Autodesk Inventor part; units mm, degrees
(part 2 of 2)
  line L937 (28.6172, -1.9519) -> (28.5556, -1.9543)
  line L938 (28.5556, -1.9543) -> (28.5008, -1.9651)
  line L939 (28.5008, -1.9651) -> (28.4534, -1.9836)
  line L940 (28.4534, -1.9836) -> (28.4139, -2.0092)
  line L941 (28.4139, -2.0092) -> (28.3764, -2.0503)
  line L942 (28.3764, -2.0503) -> (28.2958, -2.1772)
  line L943 (28.2958, -2.1772) -> (28.1956, -2.3218)
  line L944 (28.1956, -2.3218) -> (28.0891, -2.4618)
  line L945 (28.0891, -2.4618) -> (27.9933, -2.5776)
  line L946 (27.9933, -2.5776) -> (27.9658, -2.626)
  line L947 (27.9658, -2.626) -> (27.9536, -2.6714)
  line L948 (27.9536, -2.6714) -> (27.9506, -2.7222)
  line L949 (27.9506, -2.7222) -> (27.9573, -2.7777)
  line L950 (27.9573, -2.7777) -> (27.974, -2.837)
  line L951 (27.974, -2.837) -> (28.001, -2.8995)
  line L952 (28.001, -2.8995) -> (28.0386, -2.9643)
  line L953 (28.0386, -2.9643) -> (28.0871, -3.0308)
  line L954 (28.0871, -3.0308) -> (28.1466, -3.098)
  line L955 (28.1466, -3.098) -> (28.2172, -3.1653)
  line L956 (28.2172, -3.1653) -> (28.2991, -3.2317)
  line L957 (28.2991, -3.2317) -> (28.3923, -3.2964)
  line L958 (28.3923, -3.2964) -> (28.4154, -3.3262)
  line L959 (28.4154, -3.3262) -> (28.4622, -3.3971)
  line L960 (28.4622, -3.3971) -> (28.5192, -3.5016)
  line L961 (28.5192, -3.5016) -> (28.5791, -3.6371)
  line L962 (28.5791, -3.6371) -> (28.6102, -3.7211)
  line L963 (28.6102, -3.7211) -> (28.6391, -3.8103)
  line L964 (28.6391, -3.8103) -> (28.6674, -3.912)
  line L965 (28.6674, -3.912) -> (28.6928, -4.0208)
  line L966 (28.6928, -4.0208) -> (28.7153, -4.1393)
  line L967 (28.7153, -4.1393) -> (28.734, -4.2669)
  line L968 (28.734, -4.2669) -> (28.7482, -4.4039)
  line L969 (28.7482, -4.4039) -> (28.7571, -4.5485)
  line L970 (28.7571, -4.5485) -> (28.7599, -4.6757)
  arc A19 (28.2849, -5.0208) -> (28.7599, -4.6757) centre (25, 0) ccw
  line L971 (28.2849, -5.0208) -> (28.1648, -4.9789)
  line L972 (28.1648, -4.9789) -> (28.0301, -4.9258)
  line L973 (28.0301, -4.9258) -> (27.9042, -4.8699)
  line L974 (27.9042, -4.8699) -> (27.7886, -4.8127)
  line L975 (27.7886, -4.8127) -> (27.6829, -4.7547)
  line L976 (27.6829, -4.7547) -> (27.5872, -4.697)
  line L977 (27.5872, -4.697) -> (27.4992, -4.6386)
  line L978 (27.4992, -4.6386) -> (27.4233, -4.5836)
  line L979 (27.4233, -4.5836) -> (27.353, -4.528)
  line L980 (27.353, -4.528) -> (27.2426, -4.4291)
  line L981 (27.2426, -4.4291) -> (27.1609, -4.3427)
  line L982 (27.1609, -4.3427) -> (27.1079, -4.2763)
  line L983 (27.1079, -4.2763) -> (27.0867, -4.2451)
  line L984 (27.0867, -4.2451) -> (27.0539, -4.1365)
  line L985 (27.0539, -4.1365) -> (27.0161, -4.0381)
  line L986 (27.0161, -4.0381) -> (26.974, -3.9501)
  line L987 (26.974, -3.9501) -> (26.9284, -3.8728)
  line L988 (26.9284, -3.8728) -> (26.8802, -3.8062)
  line L989 (26.8802, -3.8062) -> (26.8301, -3.7503)
  line L990 (26.8301, -3.7503) -> (26.779, -3.7053)
  line L991 (26.779, -3.7053) -> (26.7278, -3.6711)
  line L992 (26.7278, -3.6711) -> (26.6771, -3.6476)
  line L993 (26.6771, -3.6476) -> (26.6279, -3.6347)
  line L994 (26.6279, -3.6347) -> (26.5809, -3.6323)
  line L995 (26.5809, -3.6323) -> (26.5264, -3.6435)
  line L996 (26.5264, -3.6435) -> (26.3866, -3.6988)
  line L997 (26.3866, -3.6988) -> (26.2206, -3.7568)
  line L998 (26.2206, -3.7568) -> (26.0521, -3.8075)
  line L999 (26.0521, -3.8075) -> (25.9065, -3.8449)
  line L1000 (25.9065, -3.8449) -> (25.8559, -3.8679)
  line L1001 (25.8559, -3.8679) -> (25.8193, -3.8976)
  line L1002 (25.8193, -3.8976) -> (25.7871, -3.9369)
  line L1003 (25.7871, -3.9369) -> (25.7599, -3.9857)
  line L1004 (25.7599, -3.9857) -> (25.7385, -4.0435)
  line L1005 (25.7385, -4.0435) -> (25.7237, -4.11)
  line L1006 (25.7237, -4.11) -> (25.716, -4.1846)
  line L1007 (25.716, -4.1846) -> (25.7162, -4.2668)
  line L1008 (25.7162, -4.2668) -> (25.7248, -4.3562)
  line L1009 (25.7248, -4.3562) -> (25.7424, -4.4521)
  line L1010 (25.7424, -4.4521) -> (25.7697, -4.5539)
  line L1011 (25.7697, -4.5539) -> (25.8071, -4.6611)
  line L1012 (25.8071, -4.6611) -> (25.8082, -4.6987)
  line L1013 (25.8082, -4.6987) -> (25.8044, -4.7837)
  line L1014 (25.8044, -4.7837) -> (25.7891, -4.9016)
  line L1015 (25.7891, -4.9016) -> (25.758, -5.0465)
  line L1016 (25.758, -5.0465) -> (25.7338, -5.1328)
  line L1017 (25.7338, -5.1328) -> (25.7047, -5.2219)
  line L1018 (25.7047, -5.2219) -> (25.6678, -5.3209)
  line L1019 (25.6678, -5.3209) -> (25.6244, -5.4238)
  line L1020 (25.6244, -5.4238) -> (25.573, -5.5329)
  line L1021 (25.573, -5.5329) -> (25.5132, -5.6471)
  line L1022 (25.5132, -5.6471) -> (25.4441, -5.7663)
  line L1023 (25.4441, -5.7663) -> (25.3659, -5.8882)
  line L1024 (25.3659, -5.8882) -> (25.2934, -5.9928)
  arc A20 (24.7065, -5.9928) -> (25.2934, -5.9928) centre (25, 0) ccw
  line L1025 (24.7065, -5.9928) -> (24.634, -5.8882)
  line L1026 (24.634, -5.8882) -> (24.5563, -5.7661)
  line L1027 (24.5563, -5.7661) -> (24.4872, -5.6468)
  line L1028 (24.4872, -5.6468) -> (24.4273, -5.5326)
  line L1029 (24.4273, -5.5326) -> (24.3759, -5.4236)
  line L1030 (24.3759, -5.4236) -> (24.3325, -5.3206)
  line L1031 (24.3325, -5.3206) -> (24.2955, -5.2217)
  line L1032 (24.2955, -5.2217) -> (24.2665, -5.1326)
  line L1033 (24.2665, -5.1326) -> (24.2423, -5.0463)
  line L1034 (24.2423, -5.0463) -> (24.2111, -4.9014)
  line L1035 (24.2111, -4.9014) -> (24.1958, -4.7835)
  line L1036 (24.1958, -4.7835) -> (24.1919, -4.6986)
  line L1037 (24.1919, -4.6986) -> (24.1931, -4.6609)
  line L1038 (24.1931, -4.6609) -> (24.2304, -4.5538)
  line L1039 (24.2304, -4.5538) -> (24.2576, -4.4519)
  line L1040 (24.2576, -4.4519) -> (24.2752, -4.356)
  line L1041 (24.2752, -4.356) -> (24.2838, -4.2666)
  line L1042 (24.2838, -4.2666) -> (24.284, -4.1843)
  line L1043 (24.284, -4.1843) -> (24.2763, -4.1098)
  line L1044 (24.2763, -4.1098) -> (24.2614, -4.0433)
  line L1045 (24.2614, -4.0433) -> (24.24, -3.9855)
  line L1046 (24.24, -3.9855) -> (24.2129, -3.9368)
  line L1047 (24.2129, -3.9368) -> (24.1806, -3.8974)
  line L1048 (24.1806, -3.8974) -> (24.144, -3.8677)
  line L1049 (24.144, -3.8677) -> (24.0934, -3.8448)
  line L1050 (24.0934, -3.8448) -> (23.9478, -3.8074)
  line L1051 (23.9478, -3.8074) -> (23.7793, -3.7568)
  line L1052 (23.7793, -3.7568) -> (23.6132, -3.6988)
  line L1053 (23.6132, -3.6988) -> (23.4734, -3.6436)
  line L1054 (23.4734, -3.6436) -> (23.4189, -3.6325)
  line L1055 (23.4189, -3.6325) -> (23.3719, -3.635)
  line L1056 (23.3719, -3.635) -> (23.3227, -3.6479)
  line L1057 (23.3227, -3.6479) -> (23.272, -3.6715)
  line L1058 (23.272, -3.6715) -> (23.2208, -3.7057)
  line L1059 (23.2208, -3.7057) -> (23.1698, -3.7508)
  line L1060 (23.1698, -3.7508) -> (23.1198, -3.8066)
  line L1061 (23.1198, -3.8066) -> (23.0716, -3.8733)
  line L1062 (23.0716, -3.8733) -> (23.0261, -3.9507)
  line L1063 (23.0261, -3.9507) -> (22.984, -4.0387)
  line L1064 (22.984, -4.0387) -> (22.9463, -4.1371)
  line L1065 (22.9463, -4.1371) -> (22.9136, -4.2458)
  line L1066 (22.9136, -4.2458) -> (22.8924, -4.2769)
  line L1067 (22.8924, -4.2769) -> (22.8394, -4.3434)
  line L1068 (22.8394, -4.3434) -> (22.7578, -4.4299)
  line L1069 (22.7578, -4.4299) -> (22.6475, -4.5289)
  line L1070 (22.6475, -4.5289) -> (22.5773, -4.5845)
  line L1071 (22.5773, -4.5845) -> (22.5014, -4.6396)
  line L1072 (22.5014, -4.6396) -> (22.4134, -4.698)
  line L1073 (22.4134, -4.698) -> (22.3178, -4.7559)
  line L1074 (22.3178, -4.7559) -> (22.2121, -4.8139)
  line L1075 (22.2121, -4.8139) -> (22.0967, -4.8712)
  line L1076 (22.0967, -4.8712) -> (21.9707, -4.9272)
  line L1077 (21.9707, -4.9272) -> (21.8364, -4.9813)
  line L1078 (21.8364, -4.9813) -> (21.7179, -5.0227)
  arc A21 (21.2401, -4.6757) -> (21.7179, -5.0227) centre (25, 0) ccw
  line L1079 (21.2401, -4.6757) -> (21.2429, -4.5485)
  point P0 (0, 0)
  constraints: 2160 end point, 280 parallel, 40 point on circle, 22 centre point, 20 concentric
extrude "Extrusion1" add sketch "Sketch1" along normal blind 7.5
sketch "Sketch2" plane through (0, 0, 0) normal (0, 0, -1) x (-1, 0, 0)
  circle A0 centre (-25, 0) radius 2 projected
  line L0 (-25, 0) -> (-21.9, 0) construction
  line L1 (-25, 0) -> (-23.45, 2.6847) construction
  line L2 (-25, 0) -> (-26.55, 2.6847) construction
  line L3 (-25, 0) -> (-28.1, 0) construction
  line L4 (-25, 0) -> (-26.55, -2.6847) construction
  line L5 (-25, 0) -> (-23.45, -2.6847) construction
  line L6 (-26.55, 2.6847) -> (-23.45, 2.6847)
  line L7 (-23.45, 2.6847) -> (-21.9, 0)
  line L8 (-26.55, 2.6847) -> (-28.1, 0)
  line L9 (-28.1, 0) -> (-26.55, -2.6847)
  line L10 (-26.55, -2.6847) -> (-23.45, -2.6847)
  line L11 (-23.45, -2.6847) -> (-21.9, 0)
  line L12 (-28.6196, 0) -> (-26.8098, 3.1347)
  line L13 (-26.8098, 3.1347) -> (-23.1902, 3.1347)
  line L14 (-23.1902, 3.1347) -> (-21.3804, 0)
  line L15 (-21.3804, 0) -> (-23.1902, -3.1347)
  line L16 (-23.1902, -3.1347) -> (-26.8098, -3.1347)
  line L17 (-26.8098, -3.1347) -> (-28.6196, 0)
  point P0 (0, 0)
  dimension "d2" = 3.1
  dimension "d5" = 360
  dimension "d9" = 0.45
  constraints: 36 end point, 3 horizontal, 2 coincident, 2 parallel, 22 other
  measures "d2" distance of L0.start L0.end
  measures "d9" distance between parallel lines of L8 L12
extrude "Extrusion2" cut sketch "Sketch2" against normal blind 8 contours A0 | L6 L7 L11 L10 L9 L8 | L12 L13 L14 L15 L16 L17
body "Solid1"
